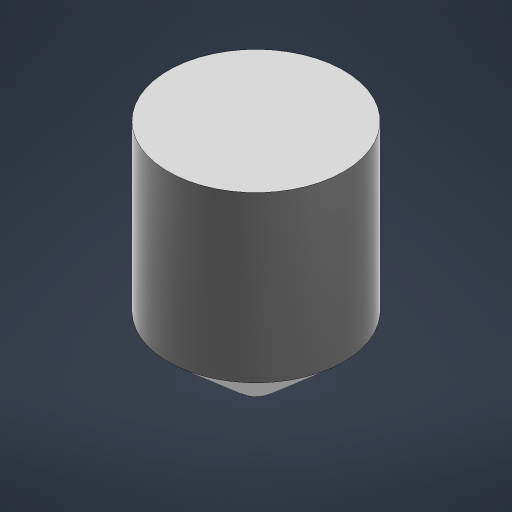
# Autodesk Inventor part: Camera_mirror
Saved by Autodesk Inventor 2024.2 (Build 282272000, 272)
## iProperties
Created: 2023-12-21
Part Number: Camera_mirror
Material: 一般
Document SubType Name: Modeling
Designer: Hanaoka
Density: 1 g/cm^3
Appearance: 既定
Author: Hanaoka
Autodesk Inventor part; units mm, degrees
ref_plane "YZ Plane" through (0, 0, 0) normal (1, 0, 0) x (0, 1, 0)
ref_plane "XZ Plane" through (0, 0, 0) normal (0, 1, 0) x (-1, 0, 0)
ref_plane "XY Plane" through (0, 0, 0) normal (0, 0, 1) x (1, 0, 0)
sketch "スケッチ1" plane through (0, 0, 0) normal (0, 0, 1) x (1, 0, 0)
  line L0 (-22.9, 20) -> (-3.9468, 3.447)
  line L1 (3.9468, 3.447) -> (22.9, 20)
  line L2 (-22.9, 20) -> (22.9, 20)
  line L3 (0, 0) -> (0, 20) construction
  line L4 (-22.9, 23) -> (22.9, 23)
  line L5 (22.9, 23) -> (22.9, 20)
  line L6 (22.9, 20) -> (-22.9, 20)
  line L7 (-22.9, 20) -> (-22.9, 23)
  line L8 (0, -407.3642) -> (0, 141.394) projected
  line L9 (0, 0) -> (0, 23)
  arc A0 (-3.9468, 3.447) -> (3.9468, 3.447) centre (0, 7.9661) ccw
  line L10 (0, -328.9702) -> (-1095, -328.9702)
  line L11 (22.9, 23) -> (25.1, 23)
  line L12 (25.1, 23) -> (25.1, 20)
  line L13 (25.1, 20) -> (26.6, 20)
  line L14 (26.6, 20) -> (26.6, 26)
  line L15 (26.6, 26) -> (-26.6, 26)
  line L16 (-26.6, 26) -> (-26.6, 20)
  line L17 (-26.6, 20) -> (-25.1, 20)
  line L18 (-25.1, 20) -> (-25.1, 23)
  line L19 (-25.1, 23) -> (-22.9, 23)
  line L20 (-22.9, 23) -> (-22.9, 63)
  line L21 (-22.9, 63) -> (22.9, 63)
  line L22 (22.9, 63) -> (22.9, 23)
  point P0 (0, 1.9661)
  point P1 (0, 26)
  point P2 (0, 63)
  dimension "d0" = 45.8
  dimension "d1" = 20
  dimension "d3" = 3
  dimension "d5" = 6
  dimension "d6" = 1095
  dimension "d8" = 2.2
  dimension "d9" = 1.5
  dimension "d10" = 3
  dimension "d14" = 40
  constraints: 44 end point, 7 perpendicular, 7 point on line, 5 horizontal, 4 parallel, 3 equal length, 2 midpoint, 2 point on circle, 2 tangent, 1 centre point, 1 coincident, 1 collinear, 1 vertical, 2 other
  measures "d0" distance of L0.start L1.end
  measures "d1" distance of L3.start L3.end
  measures "d3" distance of L6.end L4.start
  measures "d5" radius of A0
  measures "d6" distance of L10.start L10.end
  measures "d8" distance from line of L0.start L18
  measures "d9" distance of L16.end L17.end
  measures "d10" distance between parallel lines of L4 L15
  measures "d14" distance of L4.start L20.end
revolve "回転1" add sketch "スケッチ1" angle 360 about axis through (0, -10, 0) along (0, 1, 0) contours L8 L4 L5 L2 | L2 L1 A0 L8 | L8 L15 L22 L4 | L8 L21 L22 L15
